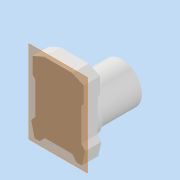
# Autodesk Inventor part: simple_lidar_shape
Saved by Autodesk Inventor 2022 (Build 260153000, 153)
## iProperties
Created: 2022-10-13
Part Number: simple_lidar_shape
Material: Générique
Document SubType Name: Modeling
Designer: andre
Density: 1 g/cm^3
Appearance: Par défaut
Author: andre
Autodesk Inventor part; units mm, degrees
ref_plane "YZ Plane" through (0, 0, 0) normal (1, 0, 0) x (0, 1, 0)
ref_plane "Plan de construction1" through (0, 0, 0) normal (0, 0, 1) x (1, 0, 0)
sketch "Esquisse1" plane through (0, 0, 0) normal (0, 0, 1) x (1, 0, 0)
  circle A0 centre (18, -9.1573) radius 3.05 projected
  arc A1 (16.3537, 35.0227) -> (19.3537, 33.6971) centre (18.8691, 36.6577) ccw projected
  arc A2 (16.3537, 35.0227) -> (9.6181, 34.9787) centre (13, 32.8427) ccw projected
  arc A3 (6.0453, 33.7654) -> (9.6181, 34.9787) centre (7.0816, 36.5807) ccw projected
  arc A4 (6.0453, 33.7654) -> (-6.0453, 33.7654) centre (0, 17.3427) ccw projected
  arc A5 (-9.6181, 34.9787) -> (-6.0453, 33.7654) centre (-7.0816, 36.5807) ccw projected
  arc A6 (-9.6181, 34.9787) -> (-16.3537, 35.0227) centre (-13, 32.8427) ccw projected
  arc A7 (-19.3537, 33.6971) -> (-16.3537, 35.0227) centre (-18.8691, 36.6577) ccw projected
  arc A8 (-19.3537, 33.6971) -> (-23.0131, 27.1188) centre (-20, 29.7497) ccw projected
  line L0 (-23.0131, 27.1188) -> (-21.6977, 25.6123) projected
  arc A9 (-21.984, 21.3792) -> (-21.6977, 25.6123) centre (-23.9573, 23.6389) ccw projected
  line L1 (-21.984, 21.3792) -> (-23.6265, 19.9451) projected
  arc A10 (-23.6265, 19.9451) -> (-23.5067, 13.8184) centre (-20.9956, 16.932) ccw projected
  arc A11 (-20.4202, 0.2907) -> (-23.5067, 13.8184) centre (-30.5395, 5.0978) ccw projected
  arc A12 (-20.4202, 0.2907) -> (-21.1202, -16.9153) centre (0, -9.1573) ccw projected
  line L2 (-21.1202, -16.9153) -> (-25.0562, -21.5766) projected
  arc A13 (-25.0562, -21.5766) -> (-25.898, -25.0549) centre (-22, -24.1573) ccw projected
  line L3 (-25.898, -25.0549) -> (-23.898, -33.7403) projected
  arc A14 (-23.898, -33.7403) -> (-16.9438, -35.4234) centre (-20, -32.8427) ccw projected
  line L4 (-16.9438, -35.4234) -> (-12.7634, -30.4726) projected
  arc A15 (-9.2394, -29.6727) -> (-12.7634, -30.4726) centre (-10.4713, -32.4081) ccw projected
  arc A16 (-9.2394, -29.6727) -> (9.2394, -29.6727) centre (0, -9.1573) ccw projected
  arc A17 (12.7634, -30.4726) -> (9.2394, -29.6727) centre (10.4713, -32.4081) ccw projected
  line L5 (12.7634, -30.4726) -> (16.9438, -35.4234) projected
  arc A18 (16.9438, -35.4234) -> (23.898, -33.7403) centre (20, -32.8427) ccw projected
  line L6 (23.898, -33.7403) -> (25.898, -25.0549) projected
  arc A19 (25.898, -25.0549) -> (25.0562, -21.5766) centre (22, -24.1573) ccw projected
  line L7 (25.0562, -21.5766) -> (21.1202, -16.9153) projected
  arc A20 (21.1202, -16.9153) -> (20.477, 0.167) centre (0, -9.1573) ccw projected
  arc A21 (23.6268, 14.7402) -> (20.477, 0.167) centre (31.8353, 5.339) ccw projected
  arc A22 (23.6268, 14.7402) -> (23.507, 20.8669) centre (20.996, 17.7533) ccw projected
  line L8 (23.507, 20.8669) -> (22.4423, 21.7255) projected
  arc A23 (22.0658, 26.0339) -> (22.4423, 21.7255) centre (24.3256, 24.0608) ccw projected
  line L9 (22.0658, 26.0339) -> (23.0131, 27.1188) projected
  arc A24 (23.0131, 27.1188) -> (19.3537, 33.6971) centre (20, 29.7497) ccw projected
  circle A25 centre (13, 32.8427) radius 2 projected
  circle A26 centre (-13, 32.8427) radius 2 projected
  circle A27 centre (-22, -24.1573) radius 2 projected
  circle A28 centre (22, -24.1573) radius 2 projected
  circle A29 centre (-18, -9.1573) radius 3.05 projected
  line L10 (0, -31.6573) -> (13.7637, -31.6573)
  line L11 (13.7637, -31.6573) -> (18.1423, -36.8427)
  line L12 (18.1423, -36.8427) -> (23.1836, -36.8427)
  line L13 (23.1836, -36.8427) -> (26.3469, -23.1052)
  line L14 (26.3469, -23.1052) -> (22.5, -18.5494)
  line L15 (22.5, -18.5494) -> (22.5, 13.6223)
  line L16 (22.5, 13.6223) -> (24.996, 16.0767)
  line L17 (24.996, 16.0767) -> (24.996, 31.9152)
  line L18 (24.996, 31.9152) -> (13.8443, 36.8427)
  line L19 (13.8443, 36.8427) -> (0, 36.8427)
  line L20 (0, 0) -> (0, -45.3526)
  line L21 (0, -31.6573) -> (-13.7637, -31.6573)
  line L22 (-13.7637, -31.6573) -> (-18.1423, -36.8427)
  line L23 (-18.1423, -36.8427) -> (-23.1836, -36.8427)
  line L24 (-23.1836, -36.8427) -> (-26.3469, -23.1052)
  line L25 (-26.3469, -23.1052) -> (-22.5, -18.5494)
  line L26 (-22.5, -18.5494) -> (-22.5, 13.6223)
  line L27 (-22.5, 13.6223) -> (-24.996, 16.0767)
  line L28 (-24.996, 16.0767) -> (-24.996, 31.9152)
  line L29 (-24.996, 31.9152) -> (-13.8443, 36.8427)
  line L30 (-13.8443, 36.8427) -> (0, 36.8427)
  point P0 (23.898, -33.7403)
  constraints: 42 end point, 9 symmetric about line, 8 tangent, 4 point on line, 3 vertical, 2 collinear, 2 horizontal, 2 point on circle, 1 perpendicular
ref_plane "Plan de construction2" through (-24.996, -18.6052, -16) normal (0, 0, -1) x (0, 1, 0)
extrude "Extrusion1" add sketch "Esquisse1" against normal up to surface (16 mm away) contours A0 | A2 L18 A24 A1 | A1 A24 L9 A23 L8 A22 A21 A20 L7 A19 L6 A18 L5 A17 A16 A15 L4 A14 L3 A13 L2 A12 A11 L26 L27 A10 L1 A9 L0 A8 A7 A6 A5 A4 A3 A2 | A2 L19 L18 | L18 L17 A22 L8 A23 L9 A24 | A2 A3 A4 A5 A6 L30 L19 | L17 L16 A22 | A6 L29 L30 | L16 A21 A22 | A6 A7 A8 L29 | L15 A20 A21 | A8 L0 A9 L1 A10 L28 L29 | L15 L7 A20 | A10 L27 L28 | L14 L13 A19 | L13 L12 A18 | A11 A12 L26 | L12 L11 A18 | A12 L2 L26 | L10 A16 A17 L5 | A13 L24 L25 | L21 L4 A15 A16 | A14 L23 L24 | L22 L23 A14 | A25 | A26 | A27 | A28 | A29
sketch "Esquisse2" plane through (0, -9.1573, -16) normal (0, 0, -1) x (-1, 0, 0)
  circle A0 centre (0, 0) radius 22.5035
  point P0 (0, 9.1573)
  constraints: 1 centre point
ref_plane "Plan de construction3" through (-23.77, -32.9273, -21) normal (0, 0, -1) x (0, 1, 0)
extrude "Extrusion2" add sketch "Esquisse2" along normal up to surface (5 mm away)
sketch "Esquisse3" plane through (0, -9.1573, -21) normal (0, 0, -1) x (-1, 0, 0)
  circle A0 centre (0, 0) radius 19.6378
  point P0 (0, 9.1573)
  constraints: 1 centre point
extrude "Extrusion3" add sketch "Esquisse3" along normal up to surface (41.2635 mm away)
